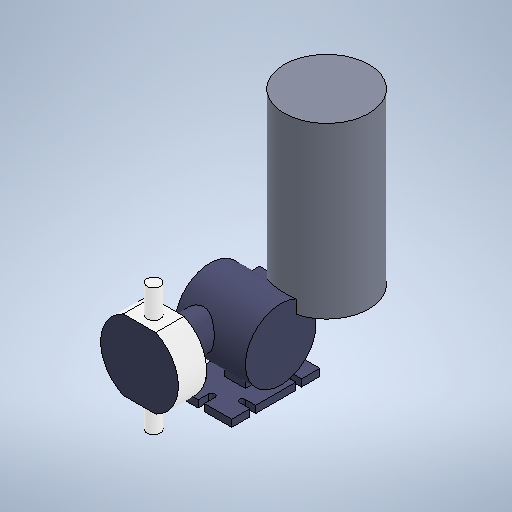
# Autodesk Inventor part: TM06198C pump
Saved by Autodesk Inventor 2025 (Build 290162010, 162A)
## iProperties
Created: 2024-11-03
Part Number: TM06198C pump
Material: Generic
Document SubType Name: Modeling
Designer: admin
Density: 1 g/cm^3
Appearance: Default
Author: admin
Autodesk Inventor part; units mm, degrees
ref_plane "YZ Plane" through (0, 0, 0) normal (1, 0, 0) x (0, 1, 0)
ref_plane "XZ Plane" through (0, 0, 0) normal (0, 1, 0) x (-1, 0, 0)
sketch "Sketch1" plane through (0, 0, 0) normal (0, 0, 1) x (1, 0, 0)
  line L0 (-43, 62.5) -> (43, 62.5)
  line L1 (43, 62.5) -> (43, -62.5)
  line L2 (43, -62.5) -> (-43, -62.5)
  line L3 (-43, -62.5) -> (-43, 62.5)
  line L4 (-43, 62.5) -> (43, -62.5) construction
  line L5 (43, 62.5) -> (-43, -62.5) construction
  line L6 (43, 36.5) -> (28, 36.5)
  arc A0 (28, 36.5) -> (28, 28.5) centre (28, 32.5) ccw
  line L7 (28, 28.5) -> (43, 28.5)
  line L8 (43, -28.5) -> (28, -28.5)
  arc A1 (28, -28.5) -> (28, -36.5) centre (28, -32.5) ccw
  line L9 (28, -36.5) -> (43, -36.5)
  line L10 (4.5, 62.5) -> (4.5, 47.5)
  arc A2 (-4.5, 47.5) -> (4.5, 47.5) centre (0, 47.5) ccw
  line L11 (-4.5, 47.5) -> (-4.5, 62.5)
  line L12 (4.5, -62.5) -> (4.5, -47.5)
  arc A3 (4.5, -47.5) -> (-4.5, -47.5) centre (0, -47.5) ccw
  line L13 (-4.5, -47.5) -> (-4.5, -62.5)
  line L14 (-43, -36.5) -> (-28, -36.5)
  arc A4 (-28, -36.5) -> (-28, -28.5) centre (-28, -32.5) ccw
  line L15 (-28, -28.5) -> (-43, -28.5)
  line L16 (-43, 28.5) -> (-28, 28.5)
  arc A5 (-28, 28.5) -> (-28, 36.5) centre (-28, 32.5) ccw
  line L17 (-28, 36.5) -> (-43, 36.5)
  line L18 (43, 0) -> (-43, 0) construction
  point P0 (0, 0)
  point P1 (0, 0)
  dimension "d0" = 86
  dimension "d1" = 125
  dimension "d2" = 4
  dimension "d3" = 65
  dimension "d4" = 15
  dimension "d5" = 4.5
  dimension "d6" = 15
  constraints: 38 end point, 16 point on line, 12 point on circle, 11 tangent, 9 perpendicular, 6 centre point, 5 midpoint, 4 equal length, 4 equal radius, 2 horizontal, 2 parallel, 2 vertical alignment, 1 horizontal alignment, 1 vertical, 1 other
  measures "d0" distance of L1.end L2.end
  measures "d1" distance of L0.end L1.end
  measures "d2" radius of A0
  measures "d3" distance of A1.centre A0.centre
  measures "d4" distance from line of L1 A0.centre
  measures "d5" radius of A2
  measures "d6" distance of L11.start L11.end
extrude "Extrusion1" add sketch "Sketch1" along normal blind 10 contours L0 L11 A2 L10 L1 L6 A0 L7 L8 A1 L9 L2 L12 A3 L13 L3 L14 A4 L15 L16 A5 L17
sketch "Sketch3" plane through (0, 0, 0) normal (0, 0, 1) x (1, 0, 0)
  line L0 (-15, 35) -> (15, 35)
  line L1 (15, 35) -> (15, -15)
  line L2 (15, -15) -> (-15, -15)
  line L3 (-15, -15) -> (-15, 35)
  point P0 (0, 0)
  point P1 (0, -15)
  dimension "d9" = 30
  dimension "d10" = 50
  dimension "d11" = 15
  constraints: 8 end point, 2 parallel, 1 horizontal, 1 midpoint, 1 perpendicular, 1 vertical alignment
  measures "d9" distance of L0.start L0.end
  measures "d10" distance of L2.end L0.start
  measures "d11" distance from line of point (0, 0) L2
extrude "Extrusion2" add sketch "Sketch3" along normal blind 120
sketch "Sketch4" plane through (0, 0, 0) normal (1, 0, 0) x (0, 1, 0)
  circle A0 centre (-20, 94) radius 50
  line L0 (28.5, 0) -> (-28.5, 0) projected
  point P0 (0, 0)
  point P1 (0, 0)
  point P2 (0, 0)
  dimension "d14" = 94
  dimension "d15" = 100
  dimension "d16" = 20
  constraints: 2 midpoint, 1 centre point
  measures "d14" vertical distance of point (0, 0) A0.centre
  measures "d15" diameter of A0
  measures "d16" horizontal distance of point (0, 0) A0.centre
extrude "Extrusion3" add sketch "Sketch4" along normal blind 70 and the other way blind 30
sketch "Sketch5" plane through (0, 0, 120) normal (0, 0, 1) x (1, 0, 0)
  circle A0 centre (55, 60) radius 60
  point P0 (0, 0)
  dimension "d21" = 120
  dimension "d22" = 55
  dimension "d23" = 60
  constraints: 1 centre point
  measures "d21" diameter of A0
  measures "d22" horizontal distance of A0.centre point (0, 0)
  measures "d23" vertical distance of A0.centre point (0, 0)
extrude "Extrusion4" add sketch "Sketch5" along normal blind 240
sketch "Sketch6" plane through (0, 0, 0) normal (0, 1, 0) x (-1, 0, 0)
  circle A0 centre (0, 100) radius 25
  point P0 (0, 0)
  dimension "d26" = 50
  dimension "d27" = 100
  constraints: 1 centre point, 1 vertical alignment
  measures "d26" diameter of A0
  measures "d27" distance of A0.centre point (0, 0)
extrude "Extrusion5" add sketch "Sketch6" against normal blind 150
sketch "Sketch7" plane through (0, -150, 100) normal (0, -1, 0) x (1, 0, 0)
  circle A0 centre (0, 0) radius 55
  line L0 (-22.9129, 50) -> (22.9129, 50)
  line L1 (-22.9129, -50) -> (22.9129, -50)
  circle A1 centre (0, 0) radius 25 construction
  line L2 (0, 0) -> (55, 0) construction
  point P0 (0, -100)
  dimension "d30" = 110
  dimension "d31" = 100
  constraints: 6 end point, 5 point on circle, 3 horizontal, 1 centre point, 1 coincident, 1 other
  measures "d30" diameter of A0
  measures "d31" distance between parallel lines of L1 L0
extrude "Extrusion6" add sketch "Sketch7" against normal blind 40 contours A0 L1 L0
ref_plane "Work Plane1" through (0, 0, 100) normal (0, 0, 1) x (1, 0, 0)
sketch "Sketch8" plane through (0, 0, 100) normal (0, 0, 1) x (1, 0, 0)
  circle A0 centre (0, -130) radius 9.525
  point P0 (0, 0)
  dimension "d35" = 19.05
  dimension "d36" = 130
  constraints: 1 centre point, 1 vertical alignment
  measures "d35" diameter of A0
  measures "d36" distance of point (0, 0) A0.centre
extrude "Extrusion7" add sketch "Sketch8" along normal mid plane 180
body "Solid1"
